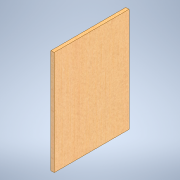
# Autodesk Inventor part: Compartment Division
Saved by Autodesk Inventor 2022.2 (Build 262287000, 287)
## iProperties
Created: 2022-02-23
Part Number: Compartment Division
Material: Pine, Southern
Document SubType Name: Modeling
Designer: PRASHANTH
Density: 0.570257 g/cm^3
Appearance: Yellow Pine - Stained Dark Medium Gloss
Author: PRASHANTH
Autodesk Inventor part; units mm, degrees
ref_plane "YZ Plane" through (0, 0, 0) normal (1, 0, 0) x (0, 1, 0)
ref_plane "XZ Plane" through (0, 0, 0) normal (0, 1, 0) x (-1, 0, 0)
ref_plane "XY Plane" through (0, 0, 0) normal (0, 0, 1) x (1, 0, 0)
sketch "Sketch1" plane through (0, 0, 0) normal (1, 0, 0) x (0, 1, 0)
  line L0 (-80, 57.5) -> (80, 57.5)
  line L1 (80, 57.5) -> (80, -57.5)
  line L2 (80, -57.5) -> (-80, -57.5)
  line L3 (-80, -57.5) -> (-80, 57.5)
  line L4 (-80, 57.5) -> (80, -57.5) construction
  line L5 (80, 57.5) -> (-80, -57.5) construction
  point P0 (0, 0)
  dimension "d0" = 160
  dimension "d1" = 115
  constraints: 12 end point, 2 midpoint, 2 parallel, 1 horizontal, 1 perpendicular
  measures "d0" distance of L1.end L2.end
  measures "d1" distance of L0.end L1.end
extrude "Extrusion1" add sketch "Sketch1" along normal blind 5
body "Solid1"
